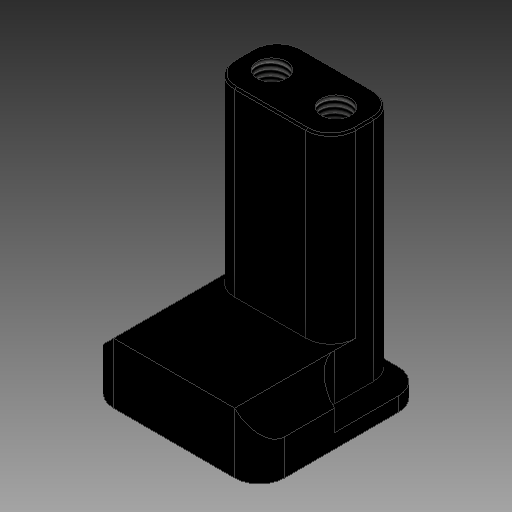
# Autodesk Inventor part: LR Rail
Saved by Autodesk Inventor 2019 (Build 230136000, 136)
## iProperties
Created: 2016-01-25
Part Number: LR Rail
Material: Aluminum 6061
Document SubType Name: Modeling
Designer: IEUser
Density: 2.7 g/cm^3
Appearance: Anodized - Black
Mass: 19.9381 g
Surface Area: 33.3973 cm^2
Volume: 7.38447 cm^3
Author: IEUser
Autodesk Inventor part; units mm, degrees
ref_plane "YZ Plane" through (0, 0, 0) normal (1, 0, 0) x (0, 1, 0)
ref_plane "XZ Plane" through (0, 0, 0) normal (0, 1, 0) x (-1, 0, 0)
ref_plane "XY Plane" through (0, 0, 0) normal (0, 0, 1) x (1, 0, 0)
sketch "Base Outline" plane through (0, 0, 0) normal (0, 1, 0) x (-1, 0, 0)
  line L0 (12, -11.5) -> (-12, -11.5)
  line L1 (-12, -11.5) -> (-12, 11.5)
  line L2 (-12, 11.5) -> (12, 11.5)
  line L3 (12, 11.5) -> (12, -11.5)
  point P0 (0, 0)
  dimension "d0" = 23
  dimension "d1" = 11.5
  dimension "d2" = 24
  dimension "d3" = 12
  constraints: 8 end point, 2 parallel, 1 horizontal, 1 perpendicular
  measures "d0" distance of L2.end L0.start
  measures "d1" distance from line of point (0, 0) L0
  measures "d2" distance of L0.start L0.end
  measures "d3" distance from line of L1 point (0, 0)
extrude "Base" add sketch "Base Outline" along normal blind 8.5
sketch "Pillar Outline" plane through (0, 8.5, 0) normal (0, 1, 0) x (1, 0, 0)
  line L0 (-8.5, 11.5) -> (8.5, 11.5)
  line L1 (8.5, 11.5) -> (8.5, 2)
  line L2 (8.5, 2) -> (-8.5, 2)
  line L3 (-8.5, 2) -> (-8.5, 11.5)
  line L4 (12, 11.5) -> (-12, 11.5) projected
  point P0 (0, 0)
  dimension "d6" = 0
  dimension "d7" = 9.5
  dimension "d8" = 17
  dimension "d9" = 8.5
  constraints: 8 end point, 2 parallel, 1 horizontal, 1 perpendicular
  measures "d6" distance between parallel lines of L4 L0
  measures "d7" distance of L2.end L0.start
  measures "d8" distance of L0.start L0.end
  measures "d9" distance from line of point (0, 0) L3
extrude "Pillar" add sketch "Pillar Outline" along normal blind 25.5
sketch "Base Cutouts Outline" plane through (0, 8.5, 0) normal (0, 1, 0) x (1, 0, 0)
  line L0 (-8.5, -1) -> (-12, -1)
  line L1 (-12, -1) -> (-12, 11.5)
  line L2 (-12, 11.5) -> (-8.5, 11.5)
  line L3 (-8.5, 11.5) -> (-8.5, -1)
  line L4 (8.5, -1) -> (12, -1)
  line L5 (12, -1) -> (12, 11.5)
  line L6 (12, 11.5) -> (8.5, 11.5)
  line L7 (8.5, 11.5) -> (8.5, -1)
  line L8 (-8.5, 11.5) -> (-12, 11.5) projected
  line L9 (-12, 11.5) -> (-12, -11.5) projected
  line L10 (-8.5, 11.5) -> (-8.5, 2) projected
  line L11 (8.5, 2) -> (8.5, 11.5) projected
  line L12 (12, 11.5) -> (8.5, 11.5) projected
  line L13 (12, -11.5) -> (12, 11.5) projected
  point P0 (0, 0)
  dimension "d12" = 0
  dimension "d13" = 0
  dimension "d14" = 0
  dimension "d15" = 12.5
  dimension "d16" = 0
  dimension "d17" = 0
  dimension "d18" = 0
  dimension "d19" = 12.5
  constraints: 16 end point, 4 parallel, 2 horizontal, 2 perpendicular
  measures "d12" distance between parallel lines of L8 L2
  measures "d13" distance between parallel lines of L9 L1
  measures "d14" distance between parallel lines of L10 L3
  measures "d15" distance of L0.end L1.end
  measures "d16" distance between parallel lines of L11 L7
  measures "d17" distance between parallel lines of L12 L6
  measures "d18" distance between parallel lines of L13 L5
  measures "d19" distance of L4.end L5.end
extrude "Base Cutouts" cut sketch "Base Cutouts Outline" against normal blind 6.5
sketch "Hole Positions" plane through (0, 34, 0) normal (0, 1, 0) x (1, 0, 0)
  line L0 (8.5, 11.5) -> (-8.5, 11.5) projected
  point P0 (0, 0)
  point P1 (4.5, 6.75)
  point P2 (-4.5, 6.75)
  dimension "d22" = 4.75
  dimension "d23" = 4.5
  dimension "d24" = 4.5
  dimension "d25" = 4.75
  measures "d22" distance from line of L0 point (4.5, 6.75)
  measures "d23" horizontal distance of point (0, 0) point (4.5, 6.75)
  measures "d24" horizontal distance of point (0, 0) point (-4.5, 6.75)
  measures "d25" distance from line of L0 point (-4.5, 6.75)
hole "Holes" at (4.5, 34, -6.75) at (-4.5, 34, -6.75) direction (0, -1, 0) diameter 4.134 depth 15 tip angle 118 thread size "M5x0.8" class "6H" standard "ISO Metric profile"
chamfer "Base Chamfer" distance 3.5 angle 45 2 edges at (-12, 8.5, 6.25) (12, 8.5, 6.25)
fillet "Pillar Fillet" radius 3.5 10 edges at (-12, 1, -11.5) (-8.5, 18, -11.5) (-8.5, 21.25, -2) (8.5, 21.25, -2) (-8.5, 5.25, 1) (-12, 2.5, 11.5) (12, 2.5, 11.5) (8.5, 5.25, 1) (12, 1, -11.5) (8.5, 18, -11.5)
chamfer "Pillar Chamfer" distance 0.25 angle 45 8 edges at (-7.4749, 34, -3.0251) (-8.5, 34, -6.75) (-7.4749, 34, -10.4749) (0, 34, -11.5) (7.4749, 34, -10.4749) (8.5, 34, -6.75) (7.4749, 34, -3.0251) (0, 34, -2)
equation "\"d1\" = 0.5 * d0"
equation "\"d3\" = 0.5 * d2"
equation "\"d9\" = 0.5 * d8"
equation "\"d19\" = d15"
equation "\"d24\" = d23"
equation "\"d25\" = d22"
body "Solid1"
